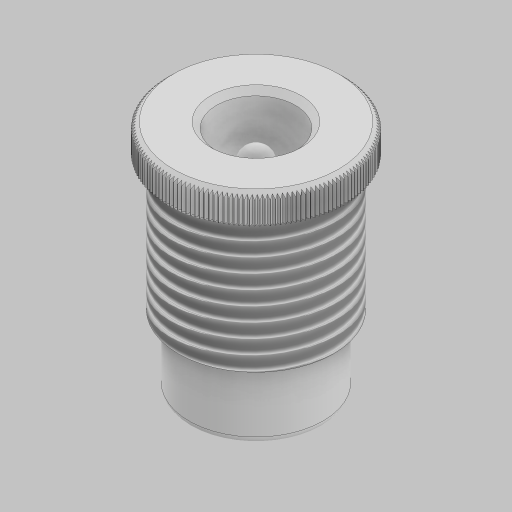
# Autodesk Inventor part: barrel-receptacle
Saved by Autodesk Inventor 2024 (Build 280153000, 153)
## iProperties
Created: 2024-11-23
Part Number: barrel-receptacle
Material: Generic
Document SubType Name: Modeling
Designer: Stefano
Density: 1 g/cm^3
Appearance: Default
Author: Stefano
Autodesk Inventor part; units mm, degrees
ref_plane "YZ Plane" through (0, 0, 0) normal (1, 0, 0) x (0, 1, 0)
ref_plane "XZ Plane" through (0, 0, 0) normal (0, 1, 0) x (-1, 0, 0)
ref_plane "XY Plane" through (0, 0, 0) normal (0, 0, 1) x (1, 0, 0)
sketch "Sketch1" plane through (0, 0, 0) normal (0, 1, 0) x (-1, 0, 0)
  circle A0 centre (0, 0) radius 6.25
  dimension "d0" = 12.5
  constraints: 1 centre point, 1 coincident
  measures "d0" diameter of A0
extrude "Extrusion1" add sketch "Sketch1" along normal blind 2
sketch "Sketch2" plane through (0, 0, 0) normal (0, -1, 0) x (1, 0, 0)
  circle A0 centre (0, 0) radius 5.5
  dimension "d3" = 11
  constraints: 1 centre point, 1 coincident
  measures "d3" diameter of A0
extrude "Extrusion2" add sketch "Sketch2" along normal blind 9.5
sketch "Sketch3" plane through (0, -9.5, 0) normal (0, -1, 0) x (1, 0, 0)
  circle A0 centre (0, 0) radius 4.75
  dimension "d6" = 9.5
  constraints: 1 centre point, 1 coincident
  measures "d6" diameter of A0
extrude "Extrusion3" add sketch "Sketch3" along normal blind 5
thread "Thread1" size "M11x1" class "6g" standard "ANSI Metric M Profile" full length
fillet "Fillet1" radius 0.5 1 edges at (-4.75, -14.5, 0)
sketch "Sketch4" plane through (0, 2, 0) normal (0, 1, 0) x (1, 0, 0)
  circle A0 centre (0, 0) radius 2.8
  dimension "d12" = 5.6
  constraints: 1 centre point, 1 coincident
  measures "d12" diameter of A0
extrude "Extrusion4" cut sketch "Sketch4" against normal blind 10.5
sketch "Sketch5" plane through (0, -8.5, 0) normal (0, 1, 0) x (1, 0, 0)
  circle A0 centre (0, 0) radius 1.05
  dimension "d15" = 2.1
  constraints: 1 centre point, 1 coincident
  measures "d15" diameter of A0
extrude "Extrusion5" add sketch "Sketch5" along normal blind 9
fillet "Fillet2" radius 1.05 1 edges at (-1.05, 0.5, 0)
sketch "Sketch6" plane through (0, 2, 0) normal (0, 1, 0) x (1, 0, 0)
  line L0 (0, 6.0489) -> (-0.1155, 6.2489)
  line L1 (0, 6.0489) -> (0.1155, 6.2489)
  line L2 (0, 0) -> (0, 6.25) construction
  circle A0 centre (0, 0) radius 6.25 projected
  dimension "d19" = 60
  dimension "d20" = 0.2
  constraints: 6 end point, 3 point on circle, 1 point on line, 1 vertical, 1 other
  measures "d19" angle of L1 L0
  measures "d20" vertical distance of L0.start L0.end
extrude "Extrusion6" cut sketch "Sketch6" against normal through all contours L0 A0 L1 picked at (-0.0513, 6.1826)
chamfer "Chamfer1" distance 0.4 angle 45 3 edges at (-2.8, 2, 0) (-4.4601, 2, -4.3784) (4.3784, 2, 4.4601)
pattern_circular "Circular Pattern1" count 150 over 360 about axis through (0, 2, 0) along (0, -1, 0) of "Extrusion6"
body "Solid1"
